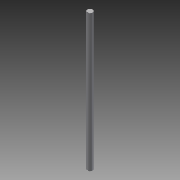
# Autodesk Inventor part: 8mm shaft
Saved by Autodesk Inventor 2013 (Build 170138000, 138)
## iProperties
Created: 2013-01-23
Part Number: 8mm shaft
Material: Steel
Document SubType Name: Modeling
Designer: actoennies
Mass: 77.1234 g
Surface Area: 55.541 cm^2
Volume: 9.82464 cm^3
Density: 7.85 g/cm^3
Author: actoennies
Autodesk Inventor part; units mm, degrees
ref_plane "YZ Plane" through (0, 0, 0) normal (1, 0, 0) x (0, 1, 0)
ref_plane "XZ Plane" through (0, 0, 0) normal (0, 1, 0) x (-1, 0, 0)
ref_plane "XY Plane" through (0, 0, 0) normal (0, 0, 1) x (1, 0, 0)
sketch "Sketch1" plane through (0, 0, 0) normal (0, 1, 0) x (-1, 0, 0)
  arc A0 (-1, 3.873) -> (1, 3.873) centre (0, 0) ccw
  line L0 (-1, 3.873) -> (-1, 3)
  line L1 (-1, 3) -> (1, 3)
  line L2 (1, 3) -> (1, 3.873)
  dimension "d0" = 8
  dimension "d1" = 2
  dimension "d2" = 1
  dimension "d3" = 1
  constraints: 6 end point, 2 point on circle, 1 centre point, 1 coincident, 1 parallel, 1 perpendicular, 1 vertical
  measures "d0" diameter of A0
  measures "d1" distance of L0.end L1.end
  measures "d2" distance edge to line of A0 L1
  measures "d3" distance from line of A0.centre L0
extrude "Extrusion1" add sketch "Sketch1" along normal blind 203.2
body "Solid1"
